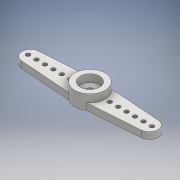
# Autodesk Inventor part: cosito servo
Saved by Autodesk Inventor 2016 (Build 200138000, 138)
## iProperties
Created: 2017-12-28
Part Number: cosito servo
Material: Genérico
Document SubType Name: Sheet Metal
Designer: David
Density: 1 g/cm^3
Sheet Metal Rule: Por defecto_mm
Appearance: Valor por defecto
Author: David
Autodesk Inventor part; units mm, degrees
ref_plane "YZ Plane" through (0, 0, 0) normal (1, 0, 0) x (0, 1, 0)
ref_plane "XZ Plane" through (0, 0, 0) normal (0, 1, 0) x (-1, 0, 0)
ref_plane "XY Plane" through (0, 0, 0) normal (0, 0, 1) x (1, 0, 0)
sketch "Boceto1" plane through (0, 0, 0) normal (0, 0, 1) x (1, 0, 0)
  arc A0 (-14.2261, 5.0309) -> (-14.2261, 1.0422) centre (-14.0761, 3.0366) ccw
  line L0 (-14.2261, 5.0309) -> (-0.0106, 6.0724)
  line L1 (-14.2261, 1.0422) -> (0, 0)
  circle A1 centre (-14.6761, 3.0366) radius 0.5
  circle A2 centre (-12.6761, 3.0366) radius 0.5
  circle A3 centre (-10.6761, 3.0366) radius 0.5
  circle A4 centre (-8.6761, 3.0366) radius 0.5
  circle A5 centre (-6.6761, 3.0366) radius 0.5
  circle A6 centre (-4.6761, 3.0366) radius 0.5
  line L2 (-0.2768, 6.0529) -> (0, 6.0731)
  arc A7 (14.2261, 1.0422) -> (14.2264, 5.0339) centre (14.0972, 3.038) ccw
  line L3 (14.2264, 5.0339) -> (0.0108, 6.0753)
  line L4 (14.2261, 1.0422) -> (0, 0)
  circle A8 centre (14.6761, 3.0366) radius 0.5
  circle A9 centre (12.6761, 3.0366) radius 0.5
  circle A10 centre (10.6761, 3.0366) radius 0.5
  circle A11 centre (8.6761, 3.0366) radius 0.5
  circle A12 centre (6.6761, 3.0366) radius 0.5
  circle A13 centre (4.6761, 3.0366) radius 0.5
  line L5 (0, 6.0731) -> (0.0201, 6.0746)
  point P0 (0, 0)
  dimension "d10" = 2
  dimension "d13" = 10
  constraints: 14 centre point, 12 end point, 4 point on circle, 3 point on line
extrude "Extrusión1" add sketch "Boceto1" along normal blind 1.6
sketch "Boceto2" plane through (0, 0, 0) normal (0, 0, -1) x (-1, 0, 0)
  line L0 (0, 0) -> (-14.2261, 1.0422) projected
  circle A0 centre (0, 3.0373) radius 3.58
  point P0 (-0.0201, 6.0746)
  constraints: 1 centre point
extrude "Extrusión2" add sketch "Boceto2" against normal blind 3.43
sketch "Boceto3" plane through (0, 0, 0) normal (0, 0, -1) x (-1, 0, 0)
  arc A0 (2.1264, 5.9174) -> (-2.122, 5.9206) centre (0, 3.0373) ccw projected
  circle A1 centre (0, 3.0373) radius 2.425
  point P0 (0, 0)
  constraints: 1 centre point, 1 coincident
extrude "Extrusión3" cut sketch "Boceto3" against normal blind 0.63
sketch "Boceto4" plane through (0, 3.0373, 0.63) normal (0, 0, -1) x (-1, 0, 0)
  circle A0 centre (0, 0) radius 0.85
  point P0 (0, -3.0373)
  constraints: 1 centre point
extrude "Extrusión4" cut sketch "Boceto4" against normal through all
sketch "Boceto5" plane through (0, 3.0373, 3.43) normal (0, 0, 1) x (1, 0, 0)
  circle A0 centre (0, 0) radius 2.3
  point P0 (0, -3.0373)
  constraints: 1 centre point
extrude "Extrusión5" cut sketch "Boceto5" against normal blind 1.83
equation "\"Radio_pliegue\" = Grosor"
equation "\"Anchura_desahogo_plegado\" = Grosor"
equation "\"Profundidad_desahogo_plegado\" = 0.5 * Grosor"
equation "\"Tamaño_destalonado\" = 4 * Grosor"
equation "\"Remanente_mínimo\" = 2 * Grosor"
equation "\"Radiodetransición\" = Radio_pliegue"
equation "\"Tamaño_de_radio_de_Jacobi\" = Radio_pliegue"
equation "\"TamañoSeparación\" = Grosor"
equation "\"Grosor\" = 0.5"
